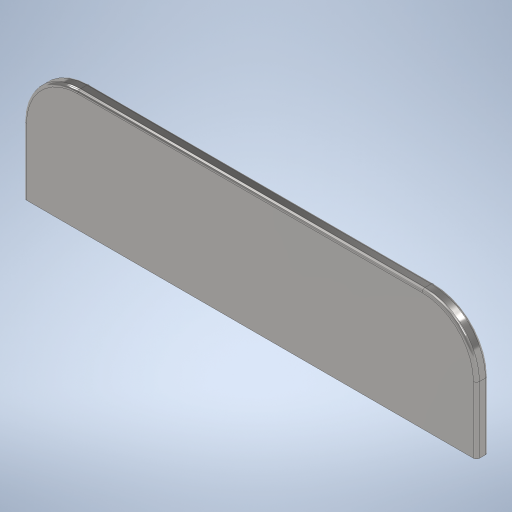
# Autodesk Inventor part: Centre Wedge
Saved by Autodesk Inventor 2024 (Build 280153000, 153)
## iProperties
Created: 2024-02-01
Part Number: Centre Wedge
Material: Generic
Document SubType Name: Modeling
Designer: HP
Density: 1 g/cm^3
Appearance: Default
Author: HP
Autodesk Inventor part; units mm, degrees
ref_plane "YZ Plane" through (0, 0, 0) normal (1, 0, 0) x (0, 1, 0)
ref_plane "XZ Plane" through (0, 0, 0) normal (0, 1, 0) x (-1, 0, 0)
ref_plane "XY Plane" through (0, 0, 0) normal (0, 0, 1) x (1, 0, 0)
sketch "Sketch1" plane through (0, 0, 0) normal (1, 0, 0) x (0, 1, 0)
  line L0 (0, 0) -> (200, 0)
  line L1 (200, 0) -> (200, 20)
  line L2 (200, 20) -> (0, 20)
  line L3 (0, 20) -> (0, 0)
  dimension "d0" = 200
  dimension "d1" = 20
  constraints: 8 end point, 2 parallel, 1 horizontal, 1 perpendicular
  measures "d0" distance of L2.end L1.end
  measures "d1" distance of L1.end L0.end
extrude "Extrusion1" add sketch "Sketch1" along normal blind 570
sketch "Sketch2" plane through (0, 0, 0) normal (0, 0, 1) x (1, 0, 0)
  line L0 (0, 200) -> (0, 0) projected
  line L1 (570, 200) -> (570, 0) projected
  line L2 (-90, 110) -> (-90, 0)
  line L3 (-90, 0) -> (0, 0)
  line L4 (0, 200) -> (0, 0)
  line L5 (570, 0) -> (570, 200)
  line L6 (660, 110) -> (660, 0)
  line L7 (660, 0) -> (570, 0)
  arc A0 (0, 200) -> (-90, 110) centre (0, 110) ccw
  arc A1 (660, 110) -> (570, 200) centre (570, 110) ccw
  point P0 (-40.5768, 141.5092)
  point P1 (615, 155)
  dimension "d11" = 90
  dimension "d12" = 90
  constraints: 12 end point, 4 point on circle, 2 centre point, 2 perpendicular, 2 vertical, 1 collinear
  measures "d11" radius of A0
  measures "d12" radius of A1
extrude "Extrusion2" add sketch "Sketch2" along normal blind 20
fillet "Fillet1" radius 5 13 edges at (-90, 55, 20) (-63.6396, 173.6396, 20) (285, 200, 20) (633.6396, 173.6396, 0) (570, 200, 10) (660, 55, 0) (660, 110, 10) (-63.6396, 173.6396, 0) (0, 200, 10) (-90, 55, 0) (-90, 110, 10) (285, 200, 0) (660, 55, 20)
body "Solid1"
